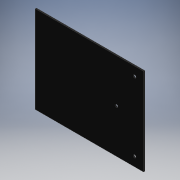
# Autodesk Inventor part: tieplate_big
Saved by Autodesk Inventor 2018 (Build 220112000, 112)
## iProperties
Created: 2017-11-16
Part Number: tieplate_big
Material: Stainless Steel
Document SubType Name: Modeling
Designer: g
Density: 8 g/cm^3
Appearance: Semi-Polished
Author: g
Autodesk Inventor part; units mm, degrees
ref_plane "YZ Plane" through (0, 0, 0) normal (1, 0, 0) x (0, 1, 0)
ref_plane "XZ Plane" through (0, 0, 0) normal (0, 1, 0) x (-1, 0, 0)
ref_plane "XY Plane" through (0, 0, 0) normal (0, 0, 1) x (1, 0, 0)
sketch "Sketch1" plane through (0, 0, 0) normal (0, 1, 0) x (-1, 0, 0)
  line L0 (0, 0) -> (180, 0)
  line L1 (180, 0) -> (180, -145)
  line L2 (180, -145) -> (0, -145)
  line L3 (0, -145) -> (0, 0)
  dimension "d0" = 180
  dimension "d1" = 145
  constraints: 8 end point, 2 parallel, 1 horizontal, 1 perpendicular
  measures "d0" distance of L1.end L2.end
  measures "d1" distance of L0.end L1.end
extrude "Extrusion1" add sketch "Sketch1" along normal blind 2
sketch "Sketch3" plane through (0, 0, 0) normal (0, -1, 0) x (1, 0, 0)
  line L0 (0, 0) -> (-15, 0) construction
  line L1 (-180, 0) -> (0, 0) projected
  line L2 (-15, 0) -> (-15, -15) construction
  circle A0 centre (-15, -15) radius 2.5
  line L3 (-180, -145) -> (-180, 0) construction
  line L4 (-180, -72.5) -> (0, -72.5) construction
  line L5 (0, 0) -> (0, -145) construction
  line L6 (0, -145) -> (-15, -145) construction
  line L7 (0, -145) -> (-180, -145) construction
  line L8 (-15, -145) -> (-15, -130) construction
  circle A1 centre (-15, -130) radius 2.5
  circle A2 centre (-45, -72.5) radius 2.5
  dimension "d4" = 15
  dimension "d5" = 15
  dimension "d6" = 5
  dimension "d7" = 15
  dimension "d8" = 5
  dimension "d9" = 5
  dimension "d10" = 45
  constraints: 10 end point, 3 centre point, 3 point on line, 2 coincident, 2 midpoint, 1 perpendicular, 1 vertical
  measures "d4" distance of L0.start L0.end
  measures "d5" distance of L0.end L2.end
  measures "d6" diameter of A0
  measures "d7" distance of L6.end L8.end
  measures "d8" diameter of A1
  measures "d9" diameter of A2
  measures "d10" distance from line of L5 A2.centre
extrude "Extrusion2" cut sketch "Sketch3" against normal blind 10
body "Solid1"
